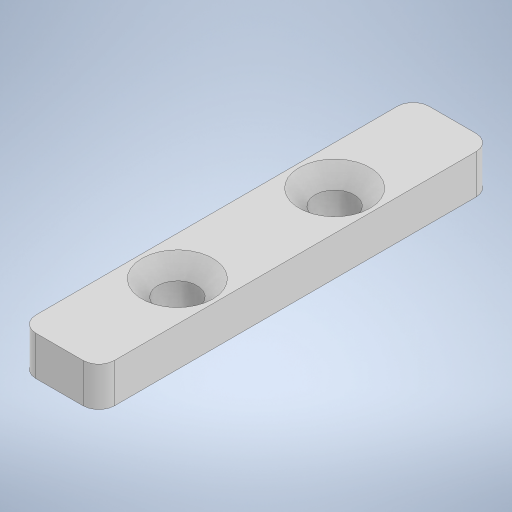
# Autodesk Inventor part: Stop
Saved by Autodesk Inventor 2023 (Build 270158000, 158)
## iProperties
Created: 2022-08-31
Part Number: Stop
Material: Generic
Document SubType Name: Modeling
Designer: ferrerx
Density: 1 g/cm^3
Appearance: Default
Author: ferrerx
Autodesk Inventor part; units mm, degrees
ref_plane "YZ Plane" through (0, 0, 0) normal (1, 0, 0) x (0, 1, 0)
ref_plane "XZ Plane" through (0, 0, 0) normal (0, 1, 0) x (-1, 0, 0)
ref_plane "XY Plane" through (0, 0, 0) normal (0, 0, 1) x (1, 0, 0)
sketch "Sketch1" plane through (0, 0, 0) normal (0, 1, 0) x (-1, 0, 0)
  line L0 (-5, 25) -> (5, 25)
  line L1 (5, 25) -> (5, -25)
  line L2 (5, -25) -> (-5, -25)
  line L3 (-5, -25) -> (-5, 25)
  line L4 (-5, 25) -> (5, -25) construction
  line L5 (5, 25) -> (-5, -25) construction
  circle A0 centre (0, 10) radius 2.5
  line L6 (0, 0) -> (5, 0) construction
  circle A1 centre (0, -10) radius 2.5
  dimension "d0" = 10
  dimension "d1" = 5
  dimension "d2" = 10
  dimension "d3" = 50
  constraints: 14 end point, 3 midpoint, 2 centre point, 2 parallel, 1 horizontal, 1 perpendicular, 1 symmetric about line, 1 other
  measures "d0" distance of L6.start A0.centre
  measures "d1" diameter of A0
  measures "d2" distance of L1.end L2.end
  measures "d3" distance of L0.end L1.end
extrude "Extrusion1" add sketch "Sketch1" along normal blind 5
fillet "Fillet1" radius 2 4 edges at (5, 2.5, 25) (5, 2.5, -25) (-5, 2.5, 25) (-5, 2.5, -25)
chamfer "Chamfer1" distance 2 angle 45 2 edges at (2.5, 5, -10) (2.5, 5, 10)
body "Solid1"
